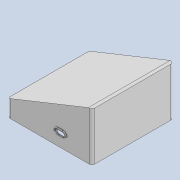
# Autodesk Inventor part: scatola - corpo - v3
Saved by Autodesk Inventor 2022 (Build 260153000, 153)
## iProperties
Created: 2025-07-11
Part Number: scatola - corpo - v3
Material: Generic
Document SubType Name: Modeling
Designer: 1234
Density: 1 g/cm^3
Appearance: Default
Author: 1234
Autodesk Inventor part; units mm, degrees
ref_plane "YZ Plane" through (0, 0, 0) normal (1, 0, 0) x (0, 1, 0)
ref_plane "XZ Plane" through (0, 0, 0) normal (0, 1, 0) x (-1, 0, 0)
ref_plane "XY Plane" through (0, 0, 0) normal (0, 0, 1) x (1, 0, 0)
sketch "Sketch1" plane through (0, 0, 0) normal (0, 0, 1) x (1, 0, 0)
  line L0 (0, 0) -> (0, 68.9891)
  line L1 (0, 68.9891) -> (-5, 68.9891)
  line L2 (-5, 68.9891) -> (-118, 23)
  line L3 (-118, 23) -> (-120, 23) construction
  line L4 (-120, 23) -> (-120, 0)
  line L5 (-120, 0) -> (0, 0)
  line L6 (-117.6086, 21) -> (-4.6086, 66.9891)
  line L7 (-4.6086, 66.9891) -> (-2, 66.9891)
  line L8 (-2, 66.9891) -> (-2, 2)
  line L9 (-2, 2) -> (-118, 2)
  line L10 (-118, 2) -> (-118, 21)
  line L11 (-118, 21) -> (-117.6086, 21)
  line L12 (-2, 2) -> (-2, 0)
  line L13 (-118, 2) -> (-118, 0)
  line L14 (-117.6086, 21) -> (-89.0038, 21) construction
  line L15 (-120, 23) -> (-5, 68.9891)
  line L16 (0.7713, 66.9891) -> (-118, 19.4918)
  point P0 (-2, 65.8809)
  dimension "d3" = 122
  dimension "d13" = 2
  dimension "d14" = 2
  dimension "d15" = 23
  dimension "d74" = 120
  dimension "d82" = 5
  dimension "d228" = 22.145
  dimension "d348" = 4
  constraints: 34 end point, 4 perpendicular, 4 point on line, 4 vertical, 2 horizontal, 1 parallel, 5 other
  measures "d3" distance of L1.end L2.end
  measures "d13" distance of L2.end L3.end
  measures "d14" distance between parallel lines of L2 L6
  measures "d15" distance of L3.end L4.end
  measures "d74" distance between parallel lines of L0 L4
  measures "d82" distance of L0.end L1.end
  measures "d228" angle of L6 L14
  measures "d348" distance between parallel lines of L15 L16
extrude "Extrusion1" add sketch "Sketch1" along normal blind 116 contours L5 L12 L8 L16 L0 | L16 L8 L7 L6 L11 L10 L13 L5 L4 L15 L1 L0 | L5 L13 L9 L12 | L16 L10 L11 L6 L7 L8
sketch "Sketch2" plane through (0, 0, 116) normal (0, 0, 1) x (1, 0, 0)
  line L0 (0, 0) -> (0, 68.9891) projected
  line L1 (0, 0) -> (0, 68.9891)
  line L2 (0, 68.9891) -> (-5, 68.9891) projected
  line L3 (0, 68.9891) -> (-5, 68.9891)
  line L4 (-120, 23) -> (-120, 0) projected
  line L5 (-120, 23) -> (-120, 0)
  line L6 (-120, 0) -> (0, 0)
  line L7 (-120, 23) -> (-5, 68.9891)
  line L8 (-48, 17.5) -> (-41, 17.5) construction
  line L9 (-48, 14) -> (-41, 14)
  line L10 (-41, 21) -> (-48, 21)
  arc A0 (-48, 21) -> (-48, 14) centre (-48, 17.5) ccw
  arc A1 (-41, 14) -> (-41, 21) centre (-41, 17.5) ccw
  point P0 (-44.5, 17.5)
  dimension "d411" = 7
  dimension "d414" = 17.5
  dimension "d415" = 41
  dimension "d416" = 3.5
  constraints: 18 end point, 4 point on circle, 4 tangent, 3 equal length, 2 centre point, 2 perpendicular, 1 horizontal, 1 midpoint
  measures "d411" distance of L8.start L8.end
  measures "d414" distance between parallel lines of L6 L8
  measures "d415" distance from line of L8.end L0
  measures "d416" radius of A1
extrude "Extrusion2" add sketch "Sketch2" against normal blind 2
sketch "Sketch3" plane through (0, 0, 0) normal (0, 0, -1) x (-1, 0, 0)
  line L0 (0, 0) -> (0, 68.9891) projected
  line L1 (0, 0) -> (0, 68.9891)
  line L2 (0, 68.9891) -> (5, 68.9891)
  line L3 (120, 23) -> (120, 0) projected
  line L4 (0, 0) -> (120, 0)
  line L5 (120, 0) -> (120, 23)
  line L6 (79, 17.5) -> (72, 17.5) construction
  line L7 (79, 14) -> (72, 14)
  line L8 (72, 21) -> (79, 21)
  arc A0 (79, 14) -> (79, 21) centre (79, 17.5) ccw
  arc A1 (72, 21) -> (72, 14) centre (72, 17.5) ccw
  line L9 (5, 68.9891) -> (120, 23) projected
  line L10 (120, 23) -> (5, 68.9891)
  point P0 (75.5, 17.5)
  dimension "d252" = 3.5
  dimension "d253" = 7
  dimension "d254" = 41
  dimension "d373" = 17.5
  constraints: 18 end point, 4 point on circle, 4 tangent, 3 equal length, 2 centre point, 2 perpendicular, 1 horizontal, 1 midpoint, 1 vertical
  measures "d252" radius of A1
  measures "d253" distance of L6.start L6.end
  measures "d254" distance from line of L3 L6.start
  measures "d373" distance between parallel lines of L4 L6
extrude "Extrusion3" add sketch "Sketch3" against normal blind 2 contours L0 L2 L9 L3 L4 | L7 A1 L8 A0
fillet "Fillet1" radius 4 4 edges at (0, 34.4946, 116) (0, 34.4946, 0) (-120, 11.5, 0) (-120, 11.5, 116)
sketch "Sketch5" plane through (-116, 0, 0) normal (0, -1, 0) x (1, 0, 0)
  circle A0 centre (0, 112) radius 4
  line L0 (0, 108) -> (-4, 108)
  line L1 (-4, 108) -> (-4, 112)
  line L2 (4, 112) -> (4, 116)
  line L3 (0, 116) -> (4, 116)
  circle A1 centre (0, 112) radius 2.3
  arc A2 (0, 116) -> (-4, 112) centre (0, 112) ccw projected
  line L4 (0, 116) -> (112, 116) projected
  line L5 (-4, 4) -> (-4, 112) projected
  line L6 (116, 4) -> (116, 112) projected
  line L7 (116, 58) -> (-26.7921, 58) construction
  line L8 (56, -9.8013) -> (56, 132.6926) construction
  line L9 (0, 0) -> (112, 0) projected
  circle A3 centre (112, 112) radius 4
  line L10 (112, 108) -> (116, 108)
  line L11 (116, 108) -> (116, 112)
  line L12 (108, 112) -> (108, 116)
  line L13 (112, 116) -> (108, 116)
  circle A4 centre (112, 112) radius 2.3
  arc A5 (116, 112) -> (112, 116) centre (112, 112) ccw
  circle A6 centre (0, 4) radius 4
  line L14 (0, 8) -> (-4, 8)
  line L15 (-4, 8) -> (-4, 4)
  line L16 (4, 4) -> (4, 0)
  line L17 (0, 0) -> (4, 0)
  circle A7 centre (0, 4) radius 2.3
  arc A8 (-4, 4) -> (0, 0) centre (0, 4) ccw
  line L18 (108, 4) -> (108, 0)
  line L19 (112, 0) -> (108, 0)
  line L20 (112, 8) -> (116, 8)
  line L21 (116, 8) -> (116, 4)
  circle A9 centre (112, 4) radius 4
  arc A10 (112, 0) -> (116, 4) centre (112, 4) ccw
  circle A11 centre (112, 4) radius 2.3
  point P0 (2, 116)
  point P1 (110, 116)
  point P2 (116, 4)
  point P3 (2, 0)
  point P4 (112, 0)
  point P5 (110, 0)
  point P6 (4, 0)
  point P7 (-4, 8)
  dimension "d58" = 4.6
  dimension "d341" = 60
  dimension "d342" = 120
  dimension "d343" = 58
  dimension "d344" = 116
  constraints: 38 symmetric about line, 36 end point, 22 point on circle, 11 centre point, 4 coincident, 3 tangent, 2 collinear, 2 horizontal, 2 midpoint, 1 concentric, 1 perpendicular, 1 vertical, 9 other
  measures "d58" diameter of A1
  measures "d341" distance between parallel lines of L5 L8
  measures "d342" distance between parallel lines of L6 L5
  measures "d343" distance between parallel lines of L9 L7
  measures "d344" distance between parallel lines of L4 L9
extrude "Extrusion5" add sketch "Sketch5" against normal blind 23 contours A0 | A0 L3 L2 | L14 A6 L5 | A6 | A6 L16 L9 | A1 | A7
ref_plane "Work Plane5" through (-2, 65.8809, 114) normal (0, -1, 0) x (1, 0, 0)
extrude "Extrusion6" add sketch "Sketch5" against normal up to surface (65.8809 mm away) contours L4 A3 L12 | A3 | L6 L10 A3 | L6 A9 L20 | L18 A9 L9 | A9 | A4 | A11
sketch "Sketch8" plane through (-116, 0, 0) normal (0, -1, 0) x (1, 0, 0)
  arc A0 (112, 7.5) -> (108.5, 4) centre (112, 4) ccw
  line L0 (116, 4) -> (116, 112) projected
  line L1 (116, 58) -> (-4, 58) construction
  line L2 (-4, 4) -> (-4, 112) projected
  line L3 (56, 58) -> (56, -13.5778) construction
  line L4 (111, 116) -> (0, 116) projected
  line L5 (106, 1.5) -> (56, 1.5)
  line L6 (114.5, 10) -> (114.5, 58)
  arc A1 (106, 1.5) -> (108.5, 4) centre (106, 4) ccw
  arc A2 (112, 7.5) -> (114.5, 10) centre (112, 10) ccw
  line L7 (112, 4) -> (56, 4) construction
  line L8 (112, 4) -> (112, 58) construction
  arc A3 (112, 0) -> (116, 4) centre (112, 4) ccw projected
  line L9 (0, 0) -> (112, 0) projected
  arc A4 (3.5, 4) -> (0, 7.5) centre (0, 4) ccw
  line L10 (6, 1.5) -> (56, 1.5)
  line L11 (-2.5, 10) -> (-2.5, 58)
  arc A5 (3.5, 4) -> (6, 1.5) centre (6, 4) ccw
  arc A6 (-2.5, 10) -> (0, 7.5) centre (0, 10) ccw
  arc A7 (108.5, 112) -> (112, 108.5) centre (112, 112) ccw
  line L12 (106, 114.5) -> (56, 114.5)
  line L13 (114.5, 106) -> (114.5, 58)
  arc A8 (108.5, 112) -> (106, 114.5) centre (106, 112) ccw
  arc A9 (114.5, 106) -> (112, 108.5) centre (112, 106) ccw
  arc A10 (0, 108.5) -> (3.5, 112) centre (0, 112) ccw
  line L14 (-2.5, 106) -> (-2.5, 58)
  line L15 (6, 114.5) -> (56, 114.5)
  arc A11 (6, 114.5) -> (3.5, 112) centre (6, 112) ccw
  arc A12 (0, 108.5) -> (-2.5, 106) centre (0, 106) ccw
  line L16 (-1, 58) -> (-1, 10)
  arc A13 (-1, 10) -> (0, 9) centre (0, 10) ccw
  arc A14 (5, 4) -> (0, 9) centre (0, 4) ccw
  arc A15 (5, 4) -> (6, 3) centre (6, 4) ccw
  line L17 (6, 3) -> (56, 3)
  line L18 (56, 3) -> (106, 3)
  arc A16 (106, 3) -> (107, 4) centre (106, 4) ccw
  arc A17 (112, 9) -> (107, 4) centre (112, 4) ccw
  arc A18 (112, 9) -> (113, 10) centre (112, 10) ccw
  line L19 (113, 10) -> (113, 58)
  line L20 (113, 58) -> (113, 106)
  arc A19 (113, 106) -> (112, 107) centre (112, 106) ccw
  arc A20 (107, 112) -> (112, 107) centre (112, 112) ccw
  arc A21 (107, 112) -> (106, 113) centre (106, 112) ccw
  line L21 (106, 113) -> (56, 113)
  line L22 (56, 113) -> (6, 113)
  arc A22 (6, 113) -> (5, 112) centre (6, 112) ccw
  arc A23 (0, 107) -> (5, 112) centre (0, 112) ccw
  arc A24 (0, 107) -> (-1, 106) centre (0, 106) ccw
  line L23 (-1, 106) -> (-1, 58)
  line L24 (56, 4.6) -> (6.5727, 4.6)
  arc A25 (6.5727, 4.6) -> (0.6, 10.5727) centre (0, 4) ccw
  line L25 (0.6, 10.5727) -> (0.6, 58)
  line L26 (0.6, 58) -> (0.6, 105.4273)
  arc A26 (0.6, 105.4273) -> (6.5727, 111.4) centre (0, 112) ccw
  line L27 (6.5727, 111.4) -> (56, 111.4)
  line L28 (56, 111.4) -> (105.4273, 111.4)
  arc A27 (105.4273, 111.4) -> (111.4, 105.4273) centre (112, 112) ccw
  line L29 (111.4, 105.4273) -> (111.4, 58)
  line L30 (111.4, 58) -> (111.4, 10.5727)
  arc A28 (111.4, 10.5727) -> (105.4273, 4.6) centre (112, 4) ccw
  line L31 (105.4273, 4.6) -> (56, 4.6)
  dimension "d286" = 3.5
  dimension "d289" = 1.5
  dimension "d290" = 1.6
  dimension "d294" = 2.5
  dimension "d295" = 2.5
  constraints: 56 end point, 56 point on circle, 28 centre point, 23 symmetric about line, 6 point on line, 4 tangent, 3 midpoint, 3 perpendicular, 2 horizontal, 1 concentric, 39 other
  measures "d286" radius of A0
  measures "d289" distance between parallel lines of L11 L16
  measures "d290" distance between parallel lines of L17 L24
  measures "d294" radius of A1
  measures "d295" radius of A2
extrude "Extrusion11" cut sketch "Sketch5" against normal blind 7 contours A1 | A4 | A7 | A11
extrude "Extrusion12" cut sketch "Sketch8" against normal blind 0.75 contours A0 A1 L5 L10 A5 A4 A6 L11 L14 A12 A10 A11 L15 L12 A8 A7 A9 L13 L6 A2
extrude "Extrusion36" cut sketch "Sketch8" against normal up to surface (2 mm away) contours L24 A25 L25 L26 A26 L27 L28 A27 L29 L30 A28 L31
ref_plane "Work Plane1" through (0, 0, 116) normal (0, 0, 1) x (1, 0, 0)
ref_plane "Work Plane3" through (0, 0, 58) normal (0, 0, -1) x (-1, 0, 0)
sketch "Sketch30" plane through (0, 0, 116) normal (0, 0, 1) x (1, 0, 0)
  arc A0 (-48, 21) -> (-48, 14) centre (-48, 17.5) ccw projected
  arc A1 (-41, 14) -> (-41, 21) centre (-41, 17.5) ccw projected
  line L0 (-48, 17.5) -> (-41, 17.5) construction
  line L1 (-48, 14) -> (-41, 14)
  line L2 (-41, 21) -> (-48, 21)
  arc A2 (-48, 21) -> (-48, 14) centre (-48, 17.5) ccw
  arc A3 (-41, 14) -> (-41, 21) centre (-41, 17.5) ccw
  line L3 (-48, 21.85) -> (-41, 21.85)
  arc A4 (-41, 13.15) -> (-41, 21.85) centre (-41, 17.5) ccw
  line L4 (-41, 13.15) -> (-48, 13.15)
  arc A5 (-48, 21.85) -> (-48, 13.15) centre (-48, 17.5) ccw
  line L5 (-41, 23.35) -> (-48, 23.35)
  arc A6 (-48, 23.35) -> (-48, 11.65) centre (-48, 17.5) ccw
  line L6 (-48, 11.65) -> (-41, 11.65)
  arc A7 (-41, 11.65) -> (-41, 23.35) centre (-41, 17.5) ccw
  line L7 (-53.85, 17.5) -> (-35.15, 17.5)
  point P0 (0, 0)
  point P1 (-44.5, 17.5)
  point P2 (-36.65, 17.5)
  point P3 (-52.35, 17.5)
  dimension "d419" = 3.5
  dimension "d420" = 8.7
  dimension "d421" = 1.5
  constraints: 18 end point, 14 point on circle, 6 centre point, 4 tangent, 3 parallel, 1 collinear, 1 horizontal, 1 midpoint, 6 other
  measures "d419" radius of A0
  measures "d420" distance between parallel lines of L3 L4
  measures "d421" distance between parallel lines of L3 L5
extrude "Extrusion44" add sketch "Sketch30" along normal blind 1.5 contours L7 A6 L5 A7 A4 L3 A5
chamfer "Chamfer17" distance 1 angle 45 3 edges at (-52.1366, 21.6366, 117.5) (-44.5, 23.35, 117.5) (-36.8634, 21.6366, 117.5)
fillet "Fillet4" radius 2.6 8 edges at (-8, 32.7407, 114) (-2, 33.9404, 108) (-8, 32.7407, 2) (-2, 33.9404, 8) (-112, 11.9456, 2) (-118, 10.7459, 8) (-118, 10.7459, 108.5359) (-112, 11.9456, 114)
extrude "Extrusion45" add sketch "Sketch8" against normal blind 3 from surface at -2 contours A0 A1 L5 L10 A5 A4 A6 L11 L14 A12 A10 A11 L15 L12 A8 A7 A9 L13 L6 A2 | L23 A24 A23 A22 L22 L21 A21 A20 A19 L20 L19 A18 A17 A16 L18 L17 A15 A14 A13 L16
chamfer "Chamfer13" distance 3.5 distance2 2.59 16 edges at (-60, 5, 114) (-111.1802, 5, 113.3202) (-113.1716, 5, 109.1716) (-117.3202, 5, 107.1802) (-118, 5, 58) (-117.3202, 5, 8.8198) (-113.1716, 5, 6.8284) (-111.1802, 5, 2.6798) (-60, 5, 2) (-8.8198, 5, 2.6798) (-6.8284, 5, 6.8284) (-2.6798, 5, 8.8198) (-2, 5, 58) (-2.6798, 5, 107.1802) (-6.8284, 5, 109.1716) (-8.8198, 5, 113.3202) measured on face at (-116.951, 5, 9.1569) measured on face at (-116.951, 5, 106.8431) measured on face at (-6.8284, 5.5, 109.1716) measured on face at (-110.8431, 5, 112.951) measured on face at (-7.182, 5, 7.182) measured on face at (-2.5, 5, 58) measured on face at (-9.1569, 5, 3.049) measured on face at (-9.1569, 5, 112.951) measured on face at (-3.049, 5, 106.8431) measured on face at (-3.049, 5, 9.1569) measured on face at (-113.1716, 5.5, 109.1716) measured on face at (-112.818, 5, 7.182) measured on face at (-60, 5, 2.5) measured on face at (-60, 5.5, 114) measured on face at (-110.8431, 5, 3.049) measured on face at (-117.5, 5, 58)
sketch "Sketch25" plane through (-5, 68.9891, 116) normal (-0.371315, 0.928507, 0) x (0.928507, 0.371315, 0)
  line L0 (0, 116) -> (-119.5468, 116) projected
  line L1 (0, 116) -> (0, 146)
  line L2 (0, 116) -> (0, 0) projected
  line L3 (0, 116) -> (-7.6014, 114)
  line L4 (-7.6014, 114) -> (-88, 114)
  line L5 (-114.0676, 114) -> (-7.6014, 114) projected
  line L6 (-88, 114) -> (-88, 146)
  line L7 (-88, 146) -> (0, 146)
  point P0 (66, 25.5)
  dimension "d374" = 30
  dimension "d375" = 88
  dimension "d387" = 7
  dimension "d388" = 3
  dimension "d390" = 30
  dimension "d395" = 25
  dimension "d382" = 30
  dimension "d384" = 3
  dimension "d389" = 25
  dimension "d410" = 26
  constraints: 10 end point, 4 point on line, 2 horizontal, 1 collinear, 1 equal length
  measures "d382" distance from line of L5 L1.start
  measures "d384" distance between parallel lines of L6 L1
  measures "d389" distance of L1.end L3.end
  measures "d410" distance between parallel lines of L7 L3
ref_plane "Work Plane6" through (-20, 0, 112) normal (1, 0, 0) x (0, 0, -1)
sketch "Sketch29" plane through (0, 0, 0) normal (0, 0, -1) x (-1, 0, 0)
  line L0 (22, 60.0367) -> (22, 34.8098) projected
  line L1 (66, 33.4429) -> (66, 42.4409) projected
  line L2 (22, 60.0367) -> (66, 42.4409)
  line L3 (66, 42.4409) -> (50.1398, 33.9356)
  line L4 (22, 34.8098) -> (66, 33.4429) projected
  line L5 (50.1398, 33.9356) -> (22, 60.0367)
  point P0 (0, 0)
  dimension "d402" = 50
  dimension "d403" = 21.051
  constraints: 6 end point, 3 point on line
  measures "d402" angle of L2 L3
  measures "d403" angle of L5 L2
body "Solid1"
